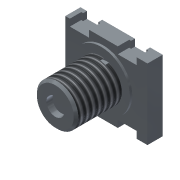
# Autodesk Inventor part: mtg flange
Saved by Autodesk Inventor 2014 (Build 180170000, 170)
## iProperties
Created: 2015-11-19
Part Number: mtg flange
Material: Generic
Document SubType Name: Modeling
Designer: Tom
Density: 1 g/cm^3
Appearance: Default
Author: Tom
Autodesk Inventor part; units mm, degrees
ref_plane "XZ Plane" through (0, 0, 0) normal (0, 1, 0) x (-1, 0, 0)
ref_plane "XY Plane" through (0, 0, 0) normal (0, 0, 1) x (1, 0, 0)
sketch "Sketch1" plane through (0, 0, 0) normal (0, 0, 1) x (1, 0, 0)
  line L0 (0, 0) -> (13.716, 0)
  line L1 (13.716, 0) -> (13.716, 11.7856)
  line L2 (13.716, 11.7856) -> (0, 11.7856)
  line L3 (0, 11.7856) -> (0, 0)
  dimension "d0" = 13.716
  dimension "d1" = 11.7856
  constraints: 8 end point, 2 parallel, 1 horizontal, 1 perpendicular
  measures "d0" distance of L2.end L1.end
  measures "d1" distance of L1.end L0.end
extrude "Extrusion1" add sketch "Sketch1" along normal blind 2.54
sketch "Sketch2" plane through (0, 0, 2.54) normal (0, 0, 1) x (1, 0, 0)
  line L0 (13.716, 0) -> (13.716, 11.7856) projected
  line L1 (13.716, 11.7856) -> (0, 11.7856) projected
  circle A0 centre (6.35, 5.8928) radius 3.4544
  dimension "d4" = 6.9088
  dimension "d5" = 7.366
  dimension "d6" = 11.7856
  dimension "d7" = 5.8928
  constraints: 1 centre point
  measures "d4" diameter of A0
  measures "d5" distance from line of L0 A0.centre
  measures "d6" distance of L0.start L0.end
  measures "d7" distance from line of L1 A0.centre
extrude "Extrusion2" add sketch "Sketch2" along normal blind 8.001
thread "Thread1" size "M7x1" class "6g" standard "ISO Metric profile" full length
sketch "Sketch3" plane through (0, 0, 2.54) normal (0, 0, 1) x (1, 0, 0)
  circle A0 centre (6.35, 5.8928) radius 3.4544 projected
  circle A1 centre (6.35, 5.8928) radius 4.826
  dimension "d12" = 9.652
  constraints: 1 centre point, 1 coincident
  measures "d12" diameter of A1
extrude "Extrusion3" add sketch "Sketch3" along normal blind 0.381
chamfer "Chamfer1" distance 0.381 angle 45 1 edges at (2.8956, 5.8928, 10.541)
ref_plane "Work Plane1" through (7.366, 0, 0) normal (1, 0, 0) x (0, 1, 0)
sketch "Sketch4" plane through (7.366, 0, 0) normal (1, 0, 0) x (0, 1, 0)
  line L0 (11.7856, 0) -> (0, 0) projected
  line L1 (9.3472, 2.921) -> (2.4384, 2.921) projected
  line L2 (5.8928, 2.921) -> (5.8928, -2.4744)
  line L3 (9.3472, 2.921) -> (9.0932, 2.921)
  line L4 (9.0932, 2.921) -> (9.0932, 3.556)
  line L5 (9.0932, 3.556) -> (9.3472, 3.556)
  line L6 (9.3472, 3.556) -> (9.3472, 2.921)
  dimension "d19" = 0.254
  dimension "d20" = 0.635
  constraints: 10 end point, 2 parallel, 2 perpendicular, 1 horizontal, 1 midpoint
  measures "d19" distance of L4.end L5.end
  measures "d20" distance of L5.end L1.start
revolve "Revolution1" cut sketch "Sketch4" angle 360 about axis through (7.366, 5.8928, 2.921) along (0, 0, -1)
sketch "Sketch5" plane through (6.35, 5.8928, 10.541) normal (0, 0, 1) x (1, 0, 0)
  circle A0 centre (0, 0) radius 4.826 projected
  circle A1 centre (0, 0) radius 1.4986
  point P0 (-6.35, -5.8928)
  dimension "d22" = 2.9972
  constraints: 1 centre point, 1 coincident
  measures "d22" diameter of A1
extrude "Extrusion4" cut sketch "Sketch5" against normal blind 1.016 contours A1
sketch "Sketch6" plane through (0, 0, 2.54) normal (0, 0, 1) x (1, 0, 0)
  line L0 (0, 0) -> (13.716, 0) projected
  line L1 (13.716, 11.7856) -> (0, 11.7856) projected
  line L2 (8.763, 0) -> (11.938, 0)
  line L3 (11.938, 0) -> (11.938, 1.143)
  line L4 (11.938, 1.143) -> (8.763, 1.143)
  line L5 (8.763, 1.143) -> (8.763, 0)
  line L6 (0.762, 0) -> (3.937, 0)
  line L7 (3.937, 0) -> (3.937, 1.143)
  line L8 (3.937, 1.143) -> (0.762, 1.143)
  line L9 (0.762, 1.143) -> (0.762, 0)
  line L10 (0.762, 11.7856) -> (3.937, 11.7856)
  line L11 (3.937, 11.7856) -> (3.937, 10.6426)
  line L12 (3.937, 10.6426) -> (0.762, 10.6426)
  line L13 (0.762, 10.6426) -> (0.762, 11.7856)
  line L14 (8.763, 11.7856) -> (11.938, 11.7856)
  line L15 (11.938, 11.7856) -> (11.938, 10.6426)
  line L16 (11.938, 10.6426) -> (8.763, 10.6426)
  line L17 (8.763, 10.6426) -> (8.763, 11.7856)
  circle A0 centre (6.35, 5.8928) radius 4.826 projected
  arc A1 (6.8134, 3.2019) -> (3.704, 6.5668) centre (6.35, 5.8928) ccw projected
  circle A2 centre (6.35, 5.8928) radius 1.4859 projected
  point P0 (11.938, 0.5715)
  point P1 (11.938, 11.2141)
  point P2 (0.762, 0.5715)
  point P3 (0.762, 11.2141)
  point P4 (2.3495, 10.6426)
  point P5 (10.3505, 10.6426)
  point P6 (2.3495, 1.143)
  point P7 (10.3505, 1.143)
  dimension "d25" = 3.175
  dimension "d26" = 3.175
  dimension "d27" = 3.175
  dimension "d28" = 3.175
  dimension "d29" = 13.716
  dimension "d30" = 11.176
  dimension "d32" = 1.143
  dimension "d33" = 1.143
  dimension "d34" = 4.826
  dimension "d35" = 0.762
  constraints: 32 end point, 8 midpoint, 8 parallel, 4 horizontal, 4 perpendicular, 4 point on line, 2 horizontal alignment, 2 vertical alignment, 1 coincident
  measures "d25" distance of L2.end L2.start
  measures "d26" distance of L6.end L6.start
  measures "d27" distance of L14.start L14.end
  measures "d28" distance of L10.start L10.end
  measures "d29" distance of L1.start L1.end
  measures "d30" distance of L2.end L6.start
  measures "d32" distance of L6.start L8.end
  measures "d33" distance of L10.start L12.end
  measures "d34" distance of L10.end L14.start
  measures "d35" distance of L0.start L6.start
extrude "Extrusion5" cut sketch "Sketch6" against normal blind 1.905 contours L9 L8 L7 L0 | L5 L4 L3 L0 | L15 L16 L17 L1 | L11 L12 L13 L1
sketch "Sketch7" plane through (0, 0, 0) normal (0, -1, 0) x (1, 0, 0)
  line L0 (3.937, 2.54) -> (3.937, 0.635) projected
  line L1 (3.937, 0.635) -> (0.762, 0.635) projected
  line L2 (0.762, 0.635) -> (0.762, 2.54) projected
  line L3 (0, 2.54) -> (0.762, 2.54) projected
  line L4 (0, 0) -> (0, 2.54) projected
  line L5 (0, 0) -> (13.716, 0) projected
  line L6 (11.938, 0.635) -> (8.763, 0.635) projected
  line L7 (8.763, 0.635) -> (8.763, 2.54) projected
  line L8 (3.937, 2.54) -> (8.763, 2.54) projected
  line L9 (11.6205, 0.635) -> (11.6205, 0)
  line L10 (8.763, 0.635) -> (11.938, 0.635) projected
  line L11 (9.0805, 0.635) -> (9.0805, 0)
  line L12 (13.716, 0) -> (0, 0) projected
  dimension "d38" = 3.175
  dimension "d39" = 2.54
  dimension "d40" = 0.3175
  constraints: 4 end point, 4 point on line, 1 parallel, 1 perpendicular
  measures "d38" distance of L6.end L6.start
  measures "d39" distance of L11.start L9.start
  measures "d40" distance of L6.start L9.start
extrude "Extrusion6" cut sketch "Sketch7" against normal up to surface (1.143 mm away) contours L6 L9 L5 L11
sketch "Sketch8" plane through (0, 0, 0) normal (0, -1, 0) x (1, 0, 0)
  line L0 (3.937, 0.635) -> (0.762, 0.635) projected
  line L1 (0, 0) -> (9.0805, 0) projected
  line L2 (1.0795, 0.635) -> (3.6195, 0.635)
  line L3 (3.6195, 0.635) -> (3.6195, 0)
  line L4 (3.6195, 0) -> (1.0795, 0)
  line L5 (1.0795, 0) -> (1.0795, 0.635)
  dimension "d43" = 2.54
  dimension "d44" = 3.175
  dimension "d45" = 0.3175
  constraints: 8 end point, 2 parallel, 2 point on line, 1 horizontal, 1 perpendicular
  measures "d43" distance of L2.start L2.end
  measures "d44" distance of L0.end L0.start
  measures "d45" distance from line of L0.end L5
extrude "Extrusion7" cut sketch "Sketch8" against normal up to surface (1.143 mm away)
sketch "Sketch9" plane through (0, 11.7856, 0) normal (0, 1, 0) x (1, 0, 0)
  line L0 (11.938, -0.635) -> (11.938, -2.54) projected
  line L1 (13.716, 0) -> (0, 0) projected
  line L2 (0.762, -0.635) -> (3.937, -0.635) projected
  line L3 (8.763, -2.54) -> (3.937, -2.54) projected
  line L4 (1.0795, -0.635) -> (3.6195, -0.635)
  line L5 (3.6195, -0.635) -> (3.6195, 0)
  line L6 (3.6195, 0) -> (1.0795, 0)
  line L7 (1.0795, 0) -> (1.0795, -0.635)
  line L8 (6.35, -2.54) -> (6.35, 1.5973)
  line L9 (11.6205, -0.635) -> (9.0805, -0.635)
  line L10 (9.0805, -0.635) -> (9.0805, 0)
  line L11 (9.0805, 0) -> (11.6205, 0)
  line L12 (11.6205, 0) -> (11.6205, -0.635)
  point P0 (12.7, 0)
  point P1 (11.938, -0.635)
  dimension "d48" = 2.54
  dimension "d49" = 3.175
  dimension "d50" = 0.3175
  dimension "d51" = 0.3175
  constraints: 18 end point, 6 symmetric about line, 2 parallel, 2 perpendicular, 2 point on line, 1 horizontal, 1 midpoint
  measures "d48" distance between parallel lines of L7 L5
  measures "d49" distance of L2.end L2.start
  measures "d50" horizontal distance of L2.start L6.end
  measures "d51" distance between parallel lines of L0 L12
extrude "Extrusion8" cut sketch "Sketch9" against normal up to surface (1.143 mm away)
equation "\"d7\" = 0.5 * d6"
equation "\"d40\" = -0.5 * d39 + 0.5 * d38"
equation "\"d45\" = -0.5 * d43 + 0.5 * d44"
equation "\"d50\" = -0.5 * d48 + 0.5 * d49"
body "Solid1"
